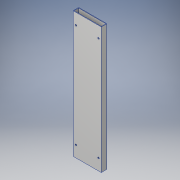
# Autodesk Inventor part: Mid
Saved by Autodesk Inventor 2019.4 (Build 234330000, 330)
## iProperties
Created: 2019-11-04
Part Number: Mid
Material: Aluminum 6061
Document SubType Name: Modeling
Designer: Mark
Density: 2.7 g/cm^3
Appearance: Aluminum - Flat
Mass: 561.254 g
Surface Area: 2088 cm^2
Volume: 207.872 cm^3
Author: Mark
Autodesk Inventor part; units mm, degrees
ref_plane "YZ Plane" through (0, 0, 0) normal (1, 0, 0) x (0, 1, 0)
ref_plane "XZ Plane" through (0, 0, 0) normal (0, 1, 0) x (-1, 0, 0)
ref_plane "XY Plane" through (0, 0, 0) normal (0, 0, 1) x (1, 0, 0)
sketch "Sketch1" plane through (0, 0, 0) normal (0, 1, 0) x (-1, 0, 0)
  line L0 (50, -10) -> (-50, -10)
  line L1 (-50, -10) -> (-50, 10)
  line L2 (-50, 10) -> (50, 10)
  line L3 (50, 10) -> (50, -10)
  line L4 (50, -10) -> (-50, 10) construction
  line L5 (-50, -10) -> (50, 10) construction
  line L6 (48, -8) -> (-48, -8)
  line L7 (-48, -8) -> (-48, 8)
  line L8 (-48, 8) -> (48, 8)
  line L9 (48, 8) -> (48, -8)
  line L10 (48, -8) -> (-48, 8) construction
  line L11 (-48, -8) -> (48, 8) construction
  point P0 (0, 0)
  dimension "d2" = 100
  dimension "d3" = 20
  dimension "d4" = 96
  dimension "d5" = 16
  constraints: 24 end point, 4 midpoint, 4 parallel, 2 horizontal, 2 perpendicular
  measures "d2" distance of L1.end L2.end
  measures "d3" distance of L0.end L1.end
  measures "d4" distance of L7.end L8.end
  measures "d5" distance of L6.end L7.end
extrude "Extrusion1" add sketch "Sketch1" along normal blind 448
sketch "Sketch2" plane through (-50, 0, 10) normal (0, 0, 1) x (1, 0, 0)
  circle A0 centre (10, 40) radius 2.75
  circle A1 centre (90, 40) radius 2.75
  circle A2 centre (10, 408) radius 2.75
  circle A3 centre (90, 408) radius 2.75
  line L0 (0, 448) -> (100, 448) projected
  line L1 (0, 0) -> (0, 448) projected
  line L2 (100, 0) -> (100, 448) projected
  line L3 (100, 0) -> (0, 0) projected
  point P0 (50, 0)
  dimension "d8" = 5.5
  dimension "d9" = 5.5
  dimension "d10" = 5.5
  dimension "d11" = 5.5
  dimension "d12" = 40
  dimension "d13" = 10
  dimension "d14" = 10
  dimension "d15" = 40
  dimension "d16" = 40
  dimension "d17" = 10
  dimension "d18" = 40
  dimension "d19" = 10
  constraints: 4 centre point
  measures "d8" diameter of A0
  measures "d9" diameter of A1
  measures "d10" diameter of A2
  measures "d11" diameter of A3
  measures "d12" distance from line of L0 A2.centre
  measures "d13" distance from line of L1 A2.centre
  measures "d14" distance from line of L2 A3.centre
  measures "d15" distance from line of L0 A3.centre
  measures "d16" distance from line of L3 A0.centre
  measures "d17" distance from line of L1 A0.centre
  measures "d18" distance from line of L3 A1.centre
  measures "d19" distance from line of L2 A1.centre
extrude "Extrusion2" cut sketch "Sketch2" against normal through all contours A0 | A1 | A2 | A3
body "Solid1"
